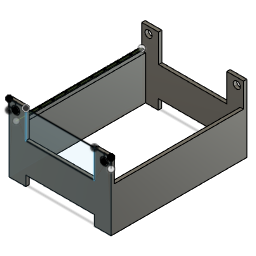
MainBody v5 (Autodesk Fusion 360 design; units mm, degrees)
description: Rack; Circular Pitch: 2.00 mm; Num Teeth: 95; Pressure Angle: 20 deg; Backlash: 0.00 mm;
Autodesk Fusion 360 part; units mm, degrees
note: some values were not read from the file. Set by a fixed rule: which sketch regions a step uses.
sketch "Sketch1" plane through (0, 0, 0) normal (0, 0, 1) x (1, 0, 0)
  line L0 (0, 0) -> (152.4, 0)
  line L1 (152.4, 0) -> (152.4, 101.6)
  line L2 (152.4, 101.6) -> (0, 101.6)
  line L3 (0, 101.6) -> (0, 0)
  line L4 (0, 0) -> (25, 0)
  line L5 (25, 15) -> (25, 0)
  line L6 (152.4, 0) -> (127.4, 0)
  line L7 (127.4, 0) -> (127.4, 15)
  line L8 (127.4, 15) -> (25, 15)
  dimension "d1" = 152.4
  dimension "d2" = 101.6
  dimension "d3" = 25
  constraint horizontal L0
  constraint vertical L1
  constraint horizontal L2
  constraint vertical L3
  constraint coincident L0.start L3.end
  constraint coincident L0 L4.end
  constraint parallel L0 L4
  constraint perpendicular L4 L5
  constraint perpendicular L1 L6
  constraint perpendicular L0 L7
  constraint perpendicular L7 L8
  measures "d1" distance of L0.start L0.end
  measures "d2" distance of L0.start L2.end
  measures "d3" distance of L0.end L6.end
extrude "Extrude1" add sketch "Sketch1" along normal blind 5 contours L0 L1 L2 L3 L4 L5 L6 L7 L8 makes body 1
sketch "Sketch2" plane through (0, 0, 0) normal (0, 0, -1) x (-1, 0, 0)
  line L0 (-152.4, 101.6) -> (-152.4, 0)
  line L1 (-152.4, 0) -> (-127.4, 0)
  line L2 (-127.4, 0) -> (-127.4, 15)
  line L3 (-127.4, 15) -> (-25, 15)
  line L4 (-25, 15) -> (-25, 0)
  line L5 (-25, 0) -> (0, 0)
  line L6 (0, 0) -> (0, 101.6)
  line L7 (0, 101.6) -> (-152.4, 101.6)
  line L8 (-152.4, 0) -> (-147.4, 0)
  line L9 (-147.4, 0) -> (-147.4, 65)
  line L10 (-147.4, 65) -> (-152.4, 65)
  line L11 (-152.4, 65) -> (-152.4, 0)
  line L12 (0, 0) -> (-6, 0)
  line L13 (-6, 0) -> (-6, 65)
  line L14 (-6, 65) -> (0, 65)
  line L15 (0, 65) -> (0, 0)
  dimension "d6" = 5
  dimension "d7" = 65
  dimension "d8" = 6
  dimension "d9" = 65
  constraint horizontal L8
  constraint vertical L9
  constraint horizontal L10
  constraint vertical L11
  constraint coincident L0.end L1.start
  constraint horizontal L12
  constraint vertical L13
  constraint horizontal L14
  constraint vertical L15
  constraint coincident L5.end L6.start
  measures "d6" distance of L0.end L8.end
  measures "d7" distance of L0.end L10.end
  measures "d8" distance of L5.end L12.end
  measures "d9" distance of L5.end L14.end
extrude "Extrude2" add sketch "Sketch2" along normal blind 193.04 contours L0 L1 L8 L9 L10 L11 | L5 L6 L12 L13 L14 L15 bodies 1
sketch "Sketch3" plane through (0, 0, -193.04) normal (0, 0, -1) x (-1, 0, 0)
  line L0 (-152.4, 65) -> (-152.4, 0)
  line L1 (-152.4, 0) -> (-147.4, 0)
  line L2 (-147.4, 0) -> (-147.4, 65)
  line L3 (-147.4, 65) -> (-152.4, 65)
  line L4 (-152.4, 0) -> (-0.3217, 0)
  line L5 (-0.3217, 0) -> (-0.3217, 101.3242)
  line L6 (-0.3217, 101.3242) -> (-152.4, 101.3242)
  line L7 (-152.4, 101.3242) -> (-152.4, 0)
  line L8 (-152.4, 0) -> (-127.4, 0)
  line L9 (-127.4, 0) -> (-127.4, 15)
  line L10 (-127.4, 15) -> (-25, 15)
  line L11 (-25, 15) -> (-25, 0)
  dimension "d12" = 25
  constraint horizontal L4
  constraint vertical L5
  constraint horizontal L6
  constraint vertical L7
  constraint coincident L0.end L1.start
  constraint perpendicular L7 L8
  constraint perpendicular L8 L9
  constraint perpendicular L9 L10
  constraint coincident L4 L11.end
  constraint perpendicular L4 L11
  measures "d12" distance of L0.end L8.end
extrude "Extrude3" add sketch "Sketch3" along normal blind 5 contours L0 L1 L2 L3 L4 L7 L8 | L2 L3 L4 L5 L6 L7 L8 L9 L10 L11 bodies 1
sketch "Sketch4" plane through (152.4, 0, 0) normal (1, 0, 0) x (0, 0, -1)
  line L0 (0, 65) -> (0, 101.6)
  line L1 (0, 101.6) -> (-5, 101.6)
  line L2 (-5, 101.6) -> (-5, 0)
  line L3 (-5, 0) -> (198.04, 0)
  line L4 (198.04, 0) -> (198.04, 101.3242)
  line L5 (198.04, 101.3242) -> (193.04, 101.3242)
  line L6 (193.04, 101.3242) -> (193.04, 65)
  line L7 (193.04, 65) -> (0, 65)
sketch "Sketch1 (2)" plane through (0, 0, 0) normal (0, 0, 1) x (1, 0, 0) in component "Rack; Circular Pitch: 2.00 mm; Num Teeth: 95; Pressure Angle: 20 deg; Backlash: 0.00 mm;"
  line L0 (-0.7839, -0.7853) -> (0, -0.5)
  line L1 (0, -0.5) -> (0.6366, -0.2683)
  line L2 (-0.7839, 0.7853) -> (0, 0.5)
  line L3 (0, 0.5) -> (0.6366, 0.2683)
  line L4 (0.6366, 0.2683) -> (0.6366, -0.2683)
  line L5 (-0.7839, 0.7853) -> (-0.7839, 1)
  line L6 (-0.7839, -0.7853) -> (-0.7839, -1)
  line L7 (-0.7839, 1.2147) -> (0, 1.5)
  line L8 (0, 1.5) -> (0.6366, 1.7317)
  line L9 (-0.7839, 2.7853) -> (0, 2.5)
  line L10 (0, 2.5) -> (0.6366, 2.2683)
  line L11 (0.6366, 2.2683) -> (0.6366, 1.7317)
  line L12 (-0.7839, 2.7853) -> (-0.7839, 3)
  line L13 (-0.7839, 1.2147) -> (-0.7839, 1)
  line L14 (-0.7839, 3.2147) -> (0, 3.5)
  line L15 (0, 3.5) -> (0.6366, 3.7317)
  line L16 (-0.7839, 4.7853) -> (0, 4.5)
  line L17 (0, 4.5) -> (0.6366, 4.2683)
  line L18 (0.6366, 4.2683) -> (0.6366, 3.7317)
  line L19 (-0.7839, 4.7853) -> (-0.7839, 5)
  line L20 (-0.7839, 3.2147) -> (-0.7839, 3)
  line L21 (-0.7839, 5.2147) -> (0, 5.5)
  line L22 (0, 5.5) -> (0.6366, 5.7317)
  line L23 (-0.7839, 6.7853) -> (0, 6.5)
  line L24 (0, 6.5) -> (0.6366, 6.2683)
  line L25 (0.6366, 6.2683) -> (0.6366, 5.7317)
  line L26 (-0.7839, 6.7853) -> (-0.7839, 7)
  line L27 (-0.7839, 5.2147) -> (-0.7839, 5)
  line L28 (-0.7839, 7.2147) -> (0, 7.5)
  line L29 (0, 7.5) -> (0.6366, 7.7317)
  line L30 (-0.7839, 8.7853) -> (0, 8.5)
  line L31 (0, 8.5) -> (0.6366, 8.2683)
  line L32 (0.6366, 8.2683) -> (0.6366, 7.7317)
  line L33 (-0.7839, 8.7853) -> (-0.7839, 9)
  line L34 (-0.7839, 7.2147) -> (-0.7839, 7)
  line L35 (-0.7839, 9.2147) -> (0, 9.5)
  line L36 (0, 9.5) -> (0.6366, 9.7317)
  line L37 (-0.7839, 10.7853) -> (0, 10.5)
  line L38 (0, 10.5) -> (0.6366, 10.2683)
  line L39 (0.6366, 10.2683) -> (0.6366, 9.7317)
  line L40 (-0.7839, 10.7853) -> (-0.7839, 11)
  line L41 (-0.7839, 9.2147) -> (-0.7839, 9)
  line L42 (-0.7839, 11.2147) -> (0, 11.5)
  line L43 (0, 11.5) -> (0.6366, 11.7317)
  line L44 (-0.7839, 12.7853) -> (0, 12.5)
  line L45 (0, 12.5) -> (0.6366, 12.2683)
  line L46 (0.6366, 12.2683) -> (0.6366, 11.7317)
  line L47 (-0.7839, 12.7853) -> (-0.7839, 13)
  line L48 (-0.7839, 11.2147) -> (-0.7839, 11)
  line L49 (-0.7839, 13.2147) -> (0, 13.5)
  line L50 (0, 13.5) -> (0.6366, 13.7317)
  line L51 (-0.7839, 14.7853) -> (0, 14.5)
  line L52 (0, 14.5) -> (0.6366, 14.2683)
  line L53 (0.6366, 14.2683) -> (0.6366, 13.7317)
  line L54 (-0.7839, 14.7853) -> (-0.7839, 15)
  line L55 (-0.7839, 13.2147) -> (-0.7839, 13)
  line L56 (-0.7839, 15.2147) -> (0, 15.5)
  line L57 (0, 15.5) -> (0.6366, 15.7317)
  line L58 (-0.7839, 16.7853) -> (0, 16.5)
  line L59 (0, 16.5) -> (0.6366, 16.2683)
  line L60 (0.6366, 16.2683) -> (0.6366, 15.7317)
  line L61 (-0.7839, 16.7853) -> (-0.7839, 17)
  line L62 (-0.7839, 15.2147) -> (-0.7839, 15)
  line L63 (-0.7839, 17.2147) -> (0, 17.5)
  line L64 (0, 17.5) -> (0.6366, 17.7317)
  line L65 (-0.7839, 18.7853) -> (0, 18.5)
  line L66 (0, 18.5) -> (0.6366, 18.2683)
  line L67 (0.6366, 18.2683) -> (0.6366, 17.7317)
  line L68 (-0.7839, 18.7853) -> (-0.7839, 19)
  line L69 (-0.7839, 17.2147) -> (-0.7839, 17)
  line L70 (-0.7839, 19.2147) -> (0, 19.5)
  line L71 (0, 19.5) -> (0.6366, 19.7317)
  line L72 (-0.7839, 20.7853) -> (0, 20.5)
  line L73 (0, 20.5) -> (0.6366, 20.2683)
  line L74 (0.6366, 20.2683) -> (0.6366, 19.7317)
  line L75 (-0.7839, 20.7853) -> (-0.7839, 21)
  line L76 (-0.7839, 19.2147) -> (-0.7839, 19)
  line L77 (-0.7839, 21.2147) -> (0, 21.5)
  line L78 (0, 21.5) -> (0.6366, 21.7317)
  line L79 (-0.7839, 22.7853) -> (0, 22.5)
  line L80 (0, 22.5) -> (0.6366, 22.2683)
  line L81 (0.6366, 22.2683) -> (0.6366, 21.7317)
  line L82 (-0.7839, 22.7853) -> (-0.7839, 23)
  line L83 (-0.7839, 21.2147) -> (-0.7839, 21)
  line L84 (-0.7839, 23.2147) -> (0, 23.5)
  line L85 (0, 23.5) -> (0.6366, 23.7317)
  line L86 (-0.7839, 24.7853) -> (0, 24.5)
  line L87 (0, 24.5) -> (0.6366, 24.2683)
  line L88 (0.6366, 24.2683) -> (0.6366, 23.7317)
  line L89 (-0.7839, 24.7853) -> (-0.7839, 25)
  line L90 (-0.7839, 23.2147) -> (-0.7839, 23)
  line L91 (-0.7839, 25.2147) -> (0, 25.5)
  line L92 (0, 25.5) -> (0.6366, 25.7317)
  line L93 (-0.7839, 26.7853) -> (0, 26.5)
  line L94 (0, 26.5) -> (0.6366, 26.2683)
  line L95 (0.6366, 26.2683) -> (0.6366, 25.7317)
  line L96 (-0.7839, 26.7853) -> (-0.7839, 27)
  line L97 (-0.7839, 25.2147) -> (-0.7839, 25)
  line L98 (-0.7839, 27.2147) -> (0, 27.5)
  line L99 (0, 27.5) -> (0.6366, 27.7317)
  line L100 (-0.7839, 28.7853) -> (0, 28.5)
  line L101 (0, 28.5) -> (0.6366, 28.2683)
  line L102 (0.6366, 28.2683) -> (0.6366, 27.7317)
  line L103 (-0.7839, 28.7853) -> (-0.7839, 29)
  line L104 (-0.7839, 27.2147) -> (-0.7839, 27)
  line L105 (-0.7839, 29.2147) -> (0, 29.5)
  line L106 (0, 29.5) -> (0.6366, 29.7317)
  line L107 (-0.7839, 30.7853) -> (0, 30.5)
  line L108 (0, 30.5) -> (0.6366, 30.2683)
  line L109 (0.6366, 30.2683) -> (0.6366, 29.7317)
  line L110 (-0.7839, 30.7853) -> (-0.7839, 31)
  line L111 (-0.7839, 29.2147) -> (-0.7839, 29)
  line L112 (-0.7839, 31.2147) -> (0, 31.5)
  line L113 (0, 31.5) -> (0.6366, 31.7317)
  line L114 (-0.7839, 32.7853) -> (0, 32.5)
  line L115 (0, 32.5) -> (0.6366, 32.2683)
  line L116 (0.6366, 32.2683) -> (0.6366, 31.7317)
  line L117 (-0.7839, 32.7853) -> (-0.7839, 33)
  line L118 (-0.7839, 31.2147) -> (-0.7839, 31)
  line L119 (-0.7839, 33.2147) -> (0, 33.5)
  line L120 (0, 33.5) -> (0.6366, 33.7317)
  line L121 (-0.7839, 34.7853) -> (0, 34.5)
  line L122 (0, 34.5) -> (0.6366, 34.2683)
  line L123 (0.6366, 34.2683) -> (0.6366, 33.7317)
  line L124 (-0.7839, 34.7853) -> (-0.7839, 35)
  line L125 (-0.7839, 33.2147) -> (-0.7839, 33)
  line L126 (-0.7839, 35.2147) -> (0, 35.5)
  line L127 (0, 35.5) -> (0.6366, 35.7317)
  line L128 (-0.7839, 36.7853) -> (0, 36.5)
  line L129 (0, 36.5) -> (0.6366, 36.2683)
  line L130 (0.6366, 36.2683) -> (0.6366, 35.7317)
  line L131 (-0.7839, 36.7853) -> (-0.7839, 37)
  line L132 (-0.7839, 35.2147) -> (-0.7839, 35)
  line L133 (-0.7839, 37.2147) -> (0, 37.5)
  line L134 (0, 37.5) -> (0.6366, 37.7317)
  line L135 (-0.7839, 38.7853) -> (0, 38.5)
  line L136 (0, 38.5) -> (0.6366, 38.2683)
  line L137 (0.6366, 38.2683) -> (0.6366, 37.7317)
  line L138 (-0.7839, 38.7853) -> (-0.7839, 39)
  line L139 (-0.7839, 37.2147) -> (-0.7839, 37)
  line L140 (-0.7839, 39.2147) -> (0, 39.5)
  line L141 (0, 39.5) -> (0.6366, 39.7317)
  line L142 (-0.7839, 40.7853) -> (0, 40.5)
  line L143 (0, 40.5) -> (0.6366, 40.2683)
  line L144 (0.6366, 40.2683) -> (0.6366, 39.7317)
  line L145 (-0.7839, 40.7853) -> (-0.7839, 41)
  line L146 (-0.7839, 39.2147) -> (-0.7839, 39)
  line L147 (-0.7839, 41.2147) -> (0, 41.5)
  line L148 (0, 41.5) -> (0.6366, 41.7317)
  line L149 (-0.7839, 42.7853) -> (0, 42.5)
  line L150 (0, 42.5) -> (0.6366, 42.2683)
  line L151 (0.6366, 42.2683) -> (0.6366, 41.7317)
  line L152 (-0.7839, 42.7853) -> (-0.7839, 43)
  line L153 (-0.7839, 41.2147) -> (-0.7839, 41)
  line L154 (-0.7839, 43.2147) -> (0, 43.5)
  line L155 (0, 43.5) -> (0.6366, 43.7317)
  line L156 (-0.7839, 44.7853) -> (0, 44.5)
  line L157 (0, 44.5) -> (0.6366, 44.2683)
  line L158 (0.6366, 44.2683) -> (0.6366, 43.7317)
  line L159 (-0.7839, 44.7853) -> (-0.7839, 45)
  line L160 (-0.7839, 43.2147) -> (-0.7839, 43)
  line L161 (-0.7839, 45.2147) -> (0, 45.5)
  line L162 (0, 45.5) -> (0.6366, 45.7317)
  line L163 (-0.7839, 46.7853) -> (0, 46.5)
  line L164 (0, 46.5) -> (0.6366, 46.2683)
  line L165 (0.6366, 46.2683) -> (0.6366, 45.7317)
  line L166 (-0.7839, 46.7853) -> (-0.7839, 47)
  line L167 (-0.7839, 45.2147) -> (-0.7839, 45)
  line L168 (-0.7839, 47.2147) -> (0, 47.5)
  line L169 (0, 47.5) -> (0.6366, 47.7317)
  line L170 (-0.7839, 48.7853) -> (0, 48.5)
  line L171 (0, 48.5) -> (0.6366, 48.2683)
  line L172 (0.6366, 48.2683) -> (0.6366, 47.7317)
  line L173 (-0.7839, 48.7853) -> (-0.7839, 49)
  line L174 (-0.7839, 47.2147) -> (-0.7839, 47)
  line L175 (-0.7839, 49.2147) -> (0, 49.5)
  line L176 (0, 49.5) -> (0.6366, 49.7317)
  line L177 (-0.7839, 50.7853) -> (0, 50.5)
  line L178 (0, 50.5) -> (0.6366, 50.2683)
  line L179 (0.6366, 50.2683) -> (0.6366, 49.7317)
  line L180 (-0.7839, 50.7853) -> (-0.7839, 51)
  line L181 (-0.7839, 49.2147) -> (-0.7839, 49)
  line L182 (-0.7839, 51.2147) -> (0, 51.5)
  line L183 (0, 51.5) -> (0.6366, 51.7317)
  line L184 (-0.7839, 52.7853) -> (0, 52.5)
  line L185 (0, 52.5) -> (0.6366, 52.2683)
  line L186 (0.6366, 52.2683) -> (0.6366, 51.7317)
  line L187 (-0.7839, 52.7853) -> (-0.7839, 53)
  line L188 (-0.7839, 51.2147) -> (-0.7839, 51)
  line L189 (-0.7839, 53.2147) -> (0, 53.5)
  line L190 (0, 53.5) -> (0.6366, 53.7317)
  line L191 (-0.7839, 54.7853) -> (0, 54.5)
  line L192 (0, 54.5) -> (0.6366, 54.2683)
  line L193 (0.6366, 54.2683) -> (0.6366, 53.7317)
  line L194 (-0.7839, 54.7853) -> (-0.7839, 55)
  line L195 (-0.7839, 53.2147) -> (-0.7839, 53)
  line L196 (-0.7839, 55.2147) -> (0, 55.5)
  line L197 (0, 55.5) -> (0.6366, 55.7317)
  line L198 (-0.7839, 56.7853) -> (0, 56.5)
  line L199 (0, 56.5) -> (0.6366, 56.2683)
  line L200 (0.6366, 56.2683) -> (0.6366, 55.7317)
  line L201 (-0.7839, 56.7853) -> (-0.7839, 57)
  line L202 (-0.7839, 55.2147) -> (-0.7839, 55)
  line L203 (-0.7839, 57.2147) -> (0, 57.5)
  line L204 (0, 57.5) -> (0.6366, 57.7317)
  line L205 (-0.7839, 58.7853) -> (0, 58.5)
  line L206 (0, 58.5) -> (0.6366, 58.2683)
  line L207 (0.6366, 58.2683) -> (0.6366, 57.7317)
  line L208 (-0.7839, 58.7853) -> (-0.7839, 59)
  line L209 (-0.7839, 57.2147) -> (-0.7839, 57)
  line L210 (-0.7839, 59.2147) -> (0, 59.5)
  line L211 (0, 59.5) -> (0.6366, 59.7317)
  line L212 (-0.7839, 60.7853) -> (0, 60.5)
  line L213 (0, 60.5) -> (0.6366, 60.2683)
  line L214 (0.6366, 60.2683) -> (0.6366, 59.7317)
  line L215 (-0.7839, 60.7853) -> (-0.7839, 61)
  line L216 (-0.7839, 59.2147) -> (-0.7839, 59)
  line L217 (-0.7839, 61.2147) -> (0, 61.5)
  line L218 (0, 61.5) -> (0.6366, 61.7317)
  line L219 (-0.7839, 62.7853) -> (0, 62.5)
  line L220 (0, 62.5) -> (0.6366, 62.2683)
  line L221 (0.6366, 62.2683) -> (0.6366, 61.7317)
  line L222 (-0.7839, 62.7853) -> (-0.7839, 63)
  line L223 (-0.7839, 61.2147) -> (-0.7839, 61)
  line L224 (-0.7839, 63.2147) -> (0, 63.5)
  line L225 (0, 63.5) -> (0.6366, 63.7317)
  line L226 (-0.7839, 64.7853) -> (0, 64.5)
  line L227 (0, 64.5) -> (0.6366, 64.2683)
  line L228 (0.6366, 64.2683) -> (0.6366, 63.7317)
  line L229 (-0.7839, 64.7853) -> (-0.7839, 65)
  line L230 (-0.7839, 63.2147) -> (-0.7839, 63)
  line L231 (-0.7839, 65.2147) -> (0, 65.5)
  line L232 (0, 65.5) -> (0.6366, 65.7317)
  line L233 (-0.7839, 66.7853) -> (0, 66.5)
  line L234 (0, 66.5) -> (0.6366, 66.2683)
  line L235 (0.6366, 66.2683) -> (0.6366, 65.7317)
  line L236 (-0.7839, 66.7853) -> (-0.7839, 67)
  line L237 (-0.7839, 65.2147) -> (-0.7839, 65)
  line L238 (-0.7839, 67.2147) -> (0, 67.5)
  line L239 (0, 67.5) -> (0.6366, 67.7317)
  line L240 (-0.7839, 68.7853) -> (0, 68.5)
  line L241 (0, 68.5) -> (0.6366, 68.2683)
  line L242 (0.6366, 68.2683) -> (0.6366, 67.7317)
  line L243 (-0.7839, 68.7853) -> (-0.7839, 69)
  line L244 (-0.7839, 67.2147) -> (-0.7839, 67)
  line L245 (-0.7839, 69.2147) -> (0, 69.5)
  line L246 (0, 69.5) -> (0.6366, 69.7317)
  line L247 (-0.7839, 70.7853) -> (0, 70.5)
  line L248 (0, 70.5) -> (0.6366, 70.2683)
  line L249 (0.6366, 70.2683) -> (0.6366, 69.7317)
  line L250 (-0.7839, 70.7853) -> (-0.7839, 71)
  line L251 (-0.7839, 69.2147) -> (-0.7839, 69)
  line L252 (-0.7839, 71.2147) -> (0, 71.5)
  line L253 (0, 71.5) -> (0.6366, 71.7317)
  line L254 (-0.7839, 72.7853) -> (0, 72.5)
  line L255 (0, 72.5) -> (0.6366, 72.2683)
  line L256 (0.6366, 72.2683) -> (0.6366, 71.7317)
  line L257 (-0.7839, 72.7853) -> (-0.7839, 73)
  line L258 (-0.7839, 71.2147) -> (-0.7839, 71)
  line L259 (-0.7839, 73.2147) -> (0, 73.5)
  line L260 (0, 73.5) -> (0.6366, 73.7317)
  line L261 (-0.7839, 74.7853) -> (0, 74.5)
  line L262 (0, 74.5) -> (0.6366, 74.2683)
  line L263 (0.6366, 74.2683) -> (0.6366, 73.7317)
  line L264 (-0.7839, 74.7853) -> (-0.7839, 75)
  line L265 (-0.7839, 73.2147) -> (-0.7839, 73)
  line L266 (-0.7839, 75.2147) -> (0, 75.5)
  line L267 (0, 75.5) -> (0.6366, 75.7317)
  line L268 (-0.7839, 76.7853) -> (0, 76.5)
  line L269 (0, 76.5) -> (0.6366, 76.2683)
  line L270 (0.6366, 76.2683) -> (0.6366, 75.7317)
  line L271 (-0.7839, 76.7853) -> (-0.7839, 77)
  line L272 (-0.7839, 75.2147) -> (-0.7839, 75)
  line L273 (-0.7839, 77.2147) -> (0, 77.5)
  line L274 (0, 77.5) -> (0.6366, 77.7317)
  line L275 (-0.7839, 78.7853) -> (0, 78.5)
  line L276 (0, 78.5) -> (0.6366, 78.2683)
  line L277 (0.6366, 78.2683) -> (0.6366, 77.7317)
  line L278 (-0.7839, 78.7853) -> (-0.7839, 79)
  line L279 (-0.7839, 77.2147) -> (-0.7839, 77)
  line L280 (-0.7839, 79.2147) -> (0, 79.5)
  line L281 (0, 79.5) -> (0.6366, 79.7317)
  line L282 (-0.7839, 80.7853) -> (0, 80.5)
  line L283 (0, 80.5) -> (0.6366, 80.2683)
  line L284 (0.6366, 80.2683) -> (0.6366, 79.7317)
  line L285 (-0.7839, 80.7853) -> (-0.7839, 81)
  line L286 (-0.7839, 79.2147) -> (-0.7839, 79)
  line L287 (-0.7839, 81.2147) -> (0, 81.5)
  line L288 (0, 81.5) -> (0.6366, 81.7317)
  line L289 (-0.7839, 82.7853) -> (0, 82.5)
  line L290 (0, 82.5) -> (0.6366, 82.2683)
  line L291 (0.6366, 82.2683) -> (0.6366, 81.7317)
  line L292 (-0.7839, 82.7853) -> (-0.7839, 83)
  line L293 (-0.7839, 81.2147) -> (-0.7839, 81)
  line L294 (-0.7839, 83.2147) -> (0, 83.5)
  line L295 (0, 83.5) -> (0.6366, 83.7317)
  line L296 (-0.7839, 84.7853) -> (0, 84.5)
  line L297 (0, 84.5) -> (0.6366, 84.2683)
  line L298 (0.6366, 84.2683) -> (0.6366, 83.7317)
  line L299 (-0.7839, 84.7853) -> (-0.7839, 85)
  line L300 (-0.7839, 83.2147) -> (-0.7839, 83)
  line L301 (-0.7839, 85.2147) -> (0, 85.5)
  line L302 (0, 85.5) -> (0.6366, 85.7317)
  line L303 (-0.7839, 86.7853) -> (0, 86.5)
  line L304 (0, 86.5) -> (0.6366, 86.2683)
  line L305 (0.6366, 86.2683) -> (0.6366, 85.7317)
  line L306 (-0.7839, 86.7853) -> (-0.7839, 87)
  line L307 (-0.7839, 85.2147) -> (-0.7839, 85)
  line L308 (-0.7839, 87.2147) -> (0, 87.5)
  line L309 (0, 87.5) -> (0.6366, 87.7317)
  line L310 (-0.7839, 88.7853) -> (0, 88.5)
  line L311 (0, 88.5) -> (0.6366, 88.2683)
  line L312 (0.6366, 88.2683) -> (0.6366, 87.7317)
  line L313 (-0.7839, 88.7853) -> (-0.7839, 89)
  line L314 (-0.7839, 87.2147) -> (-0.7839, 87)
  line L315 (-0.7839, 89.2147) -> (0, 89.5)
  line L316 (0, 89.5) -> (0.6366, 89.7317)
  line L317 (-0.7839, 90.7853) -> (0, 90.5)
  line L318 (0, 90.5) -> (0.6366, 90.2683)
  line L319 (0.6366, 90.2683) -> (0.6366, 89.7317)
  line L320 (-0.7839, 90.7853) -> (-0.7839, 91)
  line L321 (-0.7839, 89.2147) -> (-0.7839, 89)
  line L322 (-0.7839, 91.2147) -> (0, 91.5)
  line L323 (0, 91.5) -> (0.6366, 91.7317)
  line L324 (-0.7839, 92.7853) -> (0, 92.5)
  line L325 (0, 92.5) -> (0.6366, 92.2683)
  line L326 (0.6366, 92.2683) -> (0.6366, 91.7317)
  line L327 (-0.7839, 92.7853) -> (-0.7839, 93)
  line L328 (-0.7839, 91.2147) -> (-0.7839, 91)
  line L329 (-0.7839, 93.2147) -> (0, 93.5)
  line L330 (0, 93.5) -> (0.6366, 93.7317)
  line L331 (-0.7839, 94.7853) -> (0, 94.5)
  line L332 (0, 94.5) -> (0.6366, 94.2683)
  line L333 (0.6366, 94.2683) -> (0.6366, 93.7317)
  line L334 (-0.7839, 94.7853) -> (-0.7839, 95)
  line L335 (-0.7839, 93.2147) -> (-0.7839, 93)
  line L336 (-0.7839, 95.2147) -> (0, 95.5)
  line L337 (0, 95.5) -> (0.6366, 95.7317)
  line L338 (-0.7839, 96.7853) -> (0, 96.5)
  line L339 (0, 96.5) -> (0.6366, 96.2683)
  line L340 (0.6366, 96.2683) -> (0.6366, 95.7317)
  line L341 (-0.7839, 96.7853) -> (-0.7839, 97)
  line L342 (-0.7839, 95.2147) -> (-0.7839, 95)
  line L343 (-0.7839, 97.2147) -> (0, 97.5)
  line L344 (0, 97.5) -> (0.6366, 97.7317)
  line L345 (-0.7839, 98.7853) -> (0, 98.5)
  line L346 (0, 98.5) -> (0.6366, 98.2683)
  line L347 (0.6366, 98.2683) -> (0.6366, 97.7317)
  line L348 (-0.7839, 98.7853) -> (-0.7839, 99)
  line L349 (-0.7839, 97.2147) -> (-0.7839, 97)
  line L350 (-0.7839, 99.2147) -> (0, 99.5)
  line L351 (0, 99.5) -> (0.6366, 99.7317)
  line L352 (-0.7839, 100.7853) -> (0, 100.5)
  line L353 (0, 100.5) -> (0.6366, 100.2683)
  line L354 (0.6366, 100.2683) -> (0.6366, 99.7317)
  line L355 (-0.7839, 100.7853) -> (-0.7839, 101)
  line L356 (-0.7839, 99.2147) -> (-0.7839, 99)
  line L357 (-0.7839, 101.2147) -> (0, 101.5)
  line L358 (0, 101.5) -> (0.6366, 101.7317)
  line L359 (-0.7839, 102.7853) -> (0, 102.5)
  line L360 (0, 102.5) -> (0.6366, 102.2683)
  line L361 (0.6366, 102.2683) -> (0.6366, 101.7317)
  line L362 (-0.7839, 102.7853) -> (-0.7839, 103)
  line L363 (-0.7839, 101.2147) -> (-0.7839, 101)
  line L364 (-0.7839, 103.2147) -> (0, 103.5)
  line L365 (0, 103.5) -> (0.6366, 103.7317)
  line L366 (-0.7839, 104.7853) -> (0, 104.5)
  line L367 (0, 104.5) -> (0.6366, 104.2683)
  line L368 (0.6366, 104.2683) -> (0.6366, 103.7317)
  line L369 (-0.7839, 104.7853) -> (-0.7839, 105)
  line L370 (-0.7839, 103.2147) -> (-0.7839, 103)
  line L371 (-0.7839, 105.2147) -> (0, 105.5)
  line L372 (0, 105.5) -> (0.6366, 105.7317)
  line L373 (-0.7839, 106.7853) -> (0, 106.5)
  line L374 (0, 106.5) -> (0.6366, 106.2683)
  line L375 (0.6366, 106.2683) -> (0.6366, 105.7317)
  line L376 (-0.7839, 106.7853) -> (-0.7839, 107)
  line L377 (-0.7839, 105.2147) -> (-0.7839, 105)
  line L378 (-0.7839, 107.2147) -> (0, 107.5)
  line L379 (0, 107.5) -> (0.6366, 107.7317)
  line L380 (-0.7839, 108.7853) -> (0, 108.5)
  line L381 (0, 108.5) -> (0.6366, 108.2683)
  line L382 (0.6366, 108.2683) -> (0.6366, 107.7317)
  line L383 (-0.7839, 108.7853) -> (-0.7839, 109)
  line L384 (-0.7839, 107.2147) -> (-0.7839, 107)
  line L385 (-0.7839, 109.2147) -> (0, 109.5)
  line L386 (0, 109.5) -> (0.6366, 109.7317)
  line L387 (-0.7839, 110.7853) -> (0, 110.5)
  line L388 (0, 110.5) -> (0.6366, 110.2683)
  line L389 (0.6366, 110.2683) -> (0.6366, 109.7317)
  line L390 (-0.7839, 110.7853) -> (-0.7839, 111)
  line L391 (-0.7839, 109.2147) -> (-0.7839, 109)
  line L392 (-0.7839, 111.2147) -> (0, 111.5)
  line L393 (0, 111.5) -> (0.6366, 111.7317)
  line L394 (-0.7839, 112.7853) -> (0, 112.5)
  line L395 (0, 112.5) -> (0.6366, 112.2683)
  line L396 (0.6366, 112.2683) -> (0.6366, 111.7317)
  line L397 (-0.7839, 112.7853) -> (-0.7839, 113)
  line L398 (-0.7839, 111.2147) -> (-0.7839, 111)
  line L399 (-0.7839, 113.2147) -> (0, 113.5)
  line L400 (0, 113.5) -> (0.6366, 113.7317)
  line L401 (-0.7839, 114.7853) -> (0, 114.5)
  line L402 (0, 114.5) -> (0.6366, 114.2683)
  line L403 (0.6366, 114.2683) -> (0.6366, 113.7317)
  line L404 (-0.7839, 114.7853) -> (-0.7839, 115)
  line L405 (-0.7839, 113.2147) -> (-0.7839, 113)
  line L406 (-0.7839, 115.2147) -> (0, 115.5)
  line L407 (0, 115.5) -> (0.6366, 115.7317)
  line L408 (-0.7839, 116.7853) -> (0, 116.5)
  line L409 (0, 116.5) -> (0.6366, 116.2683)
  line L410 (0.6366, 116.2683) -> (0.6366, 115.7317)
  line L411 (-0.7839, 116.7853) -> (-0.7839, 117)
  line L412 (-0.7839, 115.2147) -> (-0.7839, 115)
  line L413 (-0.7839, 117.2147) -> (0, 117.5)
  line L414 (0, 117.5) -> (0.6366, 117.7317)
  line L415 (-0.7839, 118.7853) -> (0, 118.5)
  line L416 (0, 118.5) -> (0.6366, 118.2683)
  line L417 (0.6366, 118.2683) -> (0.6366, 117.7317)
  line L418 (-0.7839, 118.7853) -> (-0.7839, 119)
  line L419 (-0.7839, 117.2147) -> (-0.7839, 117)
  line L420 (-0.7839, 119.2147) -> (0, 119.5)
  line L421 (0, 119.5) -> (0.6366, 119.7317)
  line L422 (-0.7839, 120.7853) -> (0, 120.5)
  line L423 (0, 120.5) -> (0.6366, 120.2683)
  line L424 (0.6366, 120.2683) -> (0.6366, 119.7317)
  line L425 (-0.7839, 120.7853) -> (-0.7839, 121)
  line L426 (-0.7839, 119.2147) -> (-0.7839, 119)
  line L427 (-0.7839, 121.2147) -> (0, 121.5)
  line L428 (0, 121.5) -> (0.6366, 121.7317)
  line L429 (-0.7839, 122.7853) -> (0, 122.5)
  line L430 (0, 122.5) -> (0.6366, 122.2683)
  line L431 (0.6366, 122.2683) -> (0.6366, 121.7317)
  line L432 (-0.7839, 122.7853) -> (-0.7839, 123)
  line L433 (-0.7839, 121.2147) -> (-0.7839, 121)
  line L434 (-0.7839, 123.2147) -> (0, 123.5)
  line L435 (0, 123.5) -> (0.6366, 123.7317)
  line L436 (-0.7839, 124.7853) -> (0, 124.5)
  line L437 (0, 124.5) -> (0.6366, 124.2683)
  line L438 (0.6366, 124.2683) -> (0.6366, 123.7317)
  line L439 (-0.7839, 124.7853) -> (-0.7839, 125)
  line L440 (-0.7839, 123.2147) -> (-0.7839, 123)
  line L441 (-0.7839, 125.2147) -> (0, 125.5)
  line L442 (0, 125.5) -> (0.6366, 125.7317)
  line L443 (-0.7839, 126.7853) -> (0, 126.5)
  line L444 (0, 126.5) -> (0.6366, 126.2683)
  line L445 (0.6366, 126.2683) -> (0.6366, 125.7317)
  line L446 (-0.7839, 126.7853) -> (-0.7839, 127)
  line L447 (-0.7839, 125.2147) -> (-0.7839, 125)
  line L448 (-0.7839, 127.2147) -> (0, 127.5)
  line L449 (0, 127.5) -> (0.6366, 127.7317)
  line L450 (-0.7839, 128.7853) -> (0, 128.5)
  line L451 (0, 128.5) -> (0.6366, 128.2683)
  line L452 (0.6366, 128.2683) -> (0.6366, 127.7317)
  line L453 (-0.7839, 128.7853) -> (-0.7839, 129)
  line L454 (-0.7839, 127.2147) -> (-0.7839, 127)
  line L455 (-0.7839, 129.2147) -> (0, 129.5)
  line L456 (0, 129.5) -> (0.6366, 129.7317)
  line L457 (-0.7839, 130.7853) -> (0, 130.5)
  line L458 (0, 130.5) -> (0.6366, 130.2683)
  line L459 (0.6366, 130.2683) -> (0.6366, 129.7317)
  line L460 (-0.7839, 130.7853) -> (-0.7839, 131)
  line L461 (-0.7839, 129.2147) -> (-0.7839, 129)
  line L462 (-0.7839, 131.2147) -> (0, 131.5)
  line L463 (0, 131.5) -> (0.6366, 131.7317)
  line L464 (-0.7839, 132.7853) -> (0, 132.5)
  line L465 (0, 132.5) -> (0.6366, 132.2683)
  line L466 (0.6366, 132.2683) -> (0.6366, 131.7317)
  line L467 (-0.7839, 132.7853) -> (-0.7839, 133)
  line L468 (-0.7839, 131.2147) -> (-0.7839, 131)
  line L469 (-0.7839, 133.2147) -> (0, 133.5)
  line L470 (0, 133.5) -> (0.6366, 133.7317)
  line L471 (-0.7839, 134.7853) -> (0, 134.5)
  line L472 (0, 134.5) -> (0.6366, 134.2683)
  line L473 (0.6366, 134.2683) -> (0.6366, 133.7317)
  line L474 (-0.7839, 134.7853) -> (-0.7839, 135)
  line L475 (-0.7839, 133.2147) -> (-0.7839, 133)
  line L476 (-0.7839, 135.2147) -> (0, 135.5)
  line L477 (0, 135.5) -> (0.6366, 135.7317)
  line L478 (-0.7839, 136.7853) -> (0, 136.5)
  line L479 (0, 136.5) -> (0.6366, 136.2683)
  line L480 (0.6366, 136.2683) -> (0.6366, 135.7317)
  line L481 (-0.7839, 136.7853) -> (-0.7839, 137)
  line L482 (-0.7839, 135.2147) -> (-0.7839, 135)
  line L483 (-0.7839, 137.2147) -> (0, 137.5)
  line L484 (0, 137.5) -> (0.6366, 137.7317)
  line L485 (-0.7839, 138.7853) -> (0, 138.5)
  line L486 (0, 138.5) -> (0.6366, 138.2683)
  line L487 (0.6366, 138.2683) -> (0.6366, 137.7317)
  line L488 (-0.7839, 138.7853) -> (-0.7839, 139)
  line L489 (-0.7839, 137.2147) -> (-0.7839, 137)
  line L490 (-0.7839, 139.2147) -> (0, 139.5)
  line L491 (0, 139.5) -> (0.6366, 139.7317)
  line L492 (-0.7839, 140.7853) -> (0, 140.5)
  line L493 (0, 140.5) -> (0.6366, 140.2683)
  line L494 (0.6366, 140.2683) -> (0.6366, 139.7317)
  line L495 (-0.7839, 140.7853) -> (-0.7839, 141)
  line L496 (-0.7839, 139.2147) -> (-0.7839, 139)
  line L497 (-0.7839, 141.2147) -> (0, 141.5)
  line L498 (0, 141.5) -> (0.6366, 141.7317)
  line L499 (-0.7839, 142.7853) -> (0, 142.5)
  line L500 (0, 142.5) -> (0.6366, 142.2683)
  line L501 (0.6366, 142.2683) -> (0.6366, 141.7317)
  line L502 (-0.7839, 142.7853) -> (-0.7839, 143)
  line L503 (-0.7839, 141.2147) -> (-0.7839, 141)
  line L504 (-0.7839, 143.2147) -> (0, 143.5)
  line L505 (0, 143.5) -> (0.6366, 143.7317)
  line L506 (-0.7839, 144.7853) -> (0, 144.5)
  line L507 (0, 144.5) -> (0.6366, 144.2683)
  line L508 (0.6366, 144.2683) -> (0.6366, 143.7317)
  line L509 (-0.7839, 144.7853) -> (-0.7839, 145)
  line L510 (-0.7839, 143.2147) -> (-0.7839, 143)
  line L511 (-0.7839, 145.2147) -> (0, 145.5)
  line L512 (0, 145.5) -> (0.6366, 145.7317)
  line L513 (-0.7839, 146.7853) -> (0, 146.5)
  line L514 (0, 146.5) -> (0.6366, 146.2683)
  line L515 (0.6366, 146.2683) -> (0.6366, 145.7317)
  line L516 (-0.7839, 146.7853) -> (-0.7839, 147)
  line L517 (-0.7839, 145.2147) -> (-0.7839, 145)
  line L518 (-0.7839, 147.2147) -> (0, 147.5)
  line L519 (0, 147.5) -> (0.6366, 147.7317)
  line L520 (-0.7839, 148.7853) -> (0, 148.5)
  line L521 (0, 148.5) -> (0.6366, 148.2683)
  line L522 (0.6366, 148.2683) -> (0.6366, 147.7317)
  line L523 (-0.7839, 148.7853) -> (-0.7839, 149)
  line L524 (-0.7839, 147.2147) -> (-0.7839, 147)
  line L525 (-0.7839, 149.2147) -> (0, 149.5)
  line L526 (0, 149.5) -> (0.6366, 149.7317)
  line L527 (-0.7839, 150.7853) -> (0, 150.5)
  line L528 (0, 150.5) -> (0.6366, 150.2683)
  line L529 (0.6366, 150.2683) -> (0.6366, 149.7317)
  line L530 (-0.7839, 150.7853) -> (-0.7839, 151)
  line L531 (-0.7839, 149.2147) -> (-0.7839, 149)
  line L532 (-0.7839, 151.2147) -> (0, 151.5)
  line L533 (0, 151.5) -> (0.6366, 151.7317)
  line L534 (-0.7839, 152.7853) -> (0, 152.5)
  line L535 (0, 152.5) -> (0.6366, 152.2683)
  line L536 (0.6366, 152.2683) -> (0.6366, 151.7317)
  line L537 (-0.7839, 152.7853) -> (-0.7839, 153)
  line L538 (-0.7839, 151.2147) -> (-0.7839, 151)
  line L539 (-0.7839, 153.2147) -> (0, 153.5)
  line L540 (0, 153.5) -> (0.6366, 153.7317)
  line L541 (-0.7839, 154.7853) -> (0, 154.5)
  line L542 (0, 154.5) -> (0.6366, 154.2683)
  line L543 (0.6366, 154.2683) -> (0.6366, 153.7317)
  line L544 (-0.7839, 154.7853) -> (-0.7839, 155)
  line L545 (-0.7839, 153.2147) -> (-0.7839, 153)
  line L546 (-0.7839, 155.2147) -> (0, 155.5)
  line L547 (0, 155.5) -> (0.6366, 155.7317)
  line L548 (-0.7839, 156.7853) -> (0, 156.5)
  line L549 (0, 156.5) -> (0.6366, 156.2683)
  line L550 (0.6366, 156.2683) -> (0.6366, 155.7317)
  line L551 (-0.7839, 156.7853) -> (-0.7839, 157)
  line L552 (-0.7839, 155.2147) -> (-0.7839, 155)
  line L553 (-0.7839, 157.2147) -> (0, 157.5)
  line L554 (0, 157.5) -> (0.6366, 157.7317)
  line L555 (-0.7839, 158.7853) -> (0, 158.5)
  line L556 (0, 158.5) -> (0.6366, 158.2683)
  line L557 (0.6366, 158.2683) -> (0.6366, 157.7317)
  line L558 (-0.7839, 158.7853) -> (-0.7839, 159)
  line L559 (-0.7839, 157.2147) -> (-0.7839, 157)
  line L560 (-0.7839, 159.2147) -> (0, 159.5)
  line L561 (0, 159.5) -> (0.6366, 159.7317)
  line L562 (-0.7839, 160.7853) -> (0, 160.5)
  line L563 (0, 160.5) -> (0.6366, 160.2683)
  line L564 (0.6366, 160.2683) -> (0.6366, 159.7317)
  line L565 (-0.7839, 160.7853) -> (-0.7839, 161)
  line L566 (-0.7839, 159.2147) -> (-0.7839, 159)
  line L567 (-0.7839, 161.2147) -> (0, 161.5)
  line L568 (0, 161.5) -> (0.6366, 161.7317)
  line L569 (-0.7839, 162.7853) -> (0, 162.5)
  line L570 (0, 162.5) -> (0.6366, 162.2683)
  line L571 (0.6366, 162.2683) -> (0.6366, 161.7317)
  line L572 (-0.7839, 162.7853) -> (-0.7839, 163)
  line L573 (-0.7839, 161.2147) -> (-0.7839, 161)
  line L574 (-0.7839, 163.2147) -> (0, 163.5)
  line L575 (0, 163.5) -> (0.6366, 163.7317)
  line L576 (-0.7839, 164.7853) -> (0, 164.5)
  line L577 (0, 164.5) -> (0.6366, 164.2683)
  line L578 (0.6366, 164.2683) -> (0.6366, 163.7317)
  line L579 (-0.7839, 164.7853) -> (-0.7839, 165)
  line L580 (-0.7839, 163.2147) -> (-0.7839, 163)
  line L581 (-0.7839, 165.2147) -> (0, 165.5)
  line L582 (0, 165.5) -> (0.6366, 165.7317)
  line L583 (-0.7839, 166.7853) -> (0, 166.5)
  line L584 (0, 166.5) -> (0.6366, 166.2683)
  line L585 (0.6366, 166.2683) -> (0.6366, 165.7317)
  line L586 (-0.7839, 166.7853) -> (-0.7839, 167)
  line L587 (-0.7839, 165.2147) -> (-0.7839, 165)
  line L588 (-0.7839, 167.2147) -> (0, 167.5)
  line L589 (0, 167.5) -> (0.6366, 167.7317)
  line L590 (-0.7839, 168.7853) -> (0, 168.5)
  line L591 (0, 168.5) -> (0.6366, 168.2683)
  line L592 (0.6366, 168.2683) -> (0.6366, 167.7317)
  line L593 (-0.7839, 168.7853) -> (-0.7839, 169)
  line L594 (-0.7839, 167.2147) -> (-0.7839, 167)
  line L595 (-0.7839, 169.2147) -> (0, 169.5)
  line L596 (0, 169.5) -> (0.6366, 169.7317)
  line L597 (-0.7839, 170.7853) -> (0, 170.5)
  line L598 (0, 170.5) -> (0.6366, 170.2683)
  line L599 (0.6366, 170.2683) -> (0.6366, 169.7317)
  line L600 (-0.7839, 170.7853) -> (-0.7839, 171)
  line L601 (-0.7839, 169.2147) -> (-0.7839, 169)
  line L602 (-0.7839, 171.2147) -> (0, 171.5)
  line L603 (0, 171.5) -> (0.6366, 171.7317)
  line L604 (-0.7839, 172.7853) -> (0, 172.5)
  line L605 (0, 172.5) -> (0.6366, 172.2683)
  line L606 (0.6366, 172.2683) -> (0.6366, 171.7317)
  line L607 (-0.7839, 172.7853) -> (-0.7839, 173)
  line L608 (-0.7839, 171.2147) -> (-0.7839, 171)
  line L609 (-0.7839, 173.2147) -> (0, 173.5)
  line L610 (0, 173.5) -> (0.6366, 173.7317)
  line L611 (-0.7839, 174.7853) -> (0, 174.5)
  line L612 (0, 174.5) -> (0.6366, 174.2683)
  line L613 (0.6366, 174.2683) -> (0.6366, 173.7317)
  line L614 (-0.7839, 174.7853) -> (-0.7839, 175)
  line L615 (-0.7839, 173.2147) -> (-0.7839, 173)
  line L616 (-0.7839, 175.2147) -> (0, 175.5)
  line L617 (0, 175.5) -> (0.6366, 175.7317)
  line L618 (-0.7839, 176.7853) -> (0, 176.5)
  line L619 (0, 176.5) -> (0.6366, 176.2683)
  line L620 (0.6366, 176.2683) -> (0.6366, 175.7317)
  line L621 (-0.7839, 176.7853) -> (-0.7839, 177)
  line L622 (-0.7839, 175.2147) -> (-0.7839, 175)
  line L623 (-0.7839, 177.2147) -> (0, 177.5)
  line L624 (0, 177.5) -> (0.6366, 177.7317)
  line L625 (-0.7839, 178.7853) -> (0, 178.5)
  line L626 (0, 178.5) -> (0.6366, 178.2683)
  line L627 (0.6366, 178.2683) -> (0.6366, 177.7317)
  line L628 (-0.7839, 178.7853) -> (-0.7839, 179)
  line L629 (-0.7839, 177.2147) -> (-0.7839, 177)
  line L630 (-0.7839, 179.2147) -> (0, 179.5)
  line L631 (0, 179.5) -> (0.6366, 179.7317)
  line L632 (-0.7839, 180.7853) -> (0, 180.5)
  line L633 (0, 180.5) -> (0.6366, 180.2683)
  line L634 (0.6366, 180.2683) -> (0.6366, 179.7317)
  line L635 (-0.7839, 180.7853) -> (-0.7839, 181)
  line L636 (-0.7839, 179.2147) -> (-0.7839, 179)
  line L637 (-0.7839, 181.2147) -> (0, 181.5)
  line L638 (0, 181.5) -> (0.6366, 181.7317)
  line L639 (-0.7839, 182.7853) -> (0, 182.5)
  line L640 (0, 182.5) -> (0.6366, 182.2683)
  line L641 (0.6366, 182.2683) -> (0.6366, 181.7317)
  line L642 (-0.7839, 182.7853) -> (-0.7839, 183)
  line L643 (-0.7839, 181.2147) -> (-0.7839, 181)
  line L644 (-0.7839, 183.2147) -> (0, 183.5)
  line L645 (0, 183.5) -> (0.6366, 183.7317)
  line L646 (-0.7839, 184.7853) -> (0, 184.5)
  line L647 (0, 184.5) -> (0.6366, 184.2683)
  line L648 (0.6366, 184.2683) -> (0.6366, 183.7317)
  line L649 (-0.7839, 184.7853) -> (-0.7839, 185)
  line L650 (-0.7839, 183.2147) -> (-0.7839, 183)
  line L651 (-0.7839, 185.2147) -> (0, 185.5)
  line L652 (0, 185.5) -> (0.6366, 185.7317)
  line L653 (-0.7839, 186.7853) -> (0, 186.5)
  line L654 (0, 186.5) -> (0.6366, 186.2683)
  line L655 (0.6366, 186.2683) -> (0.6366, 185.7317)
  line L656 (-0.7839, 186.7853) -> (-0.7839, 187)
  line L657 (-0.7839, 185.2147) -> (-0.7839, 185)
  line L658 (-0.7839, 187.2147) -> (0, 187.5)
  line L659 (0, 187.5) -> (0.6366, 187.7317)
  line L660 (-0.7839, 188.7853) -> (0, 188.5)
  line L661 (0, 188.5) -> (0.6366, 188.2683)
  line L662 (0.6366, 188.2683) -> (0.6366, 187.7317)
  line L663 (-0.7839, 188.7853) -> (-0.7839, 189)
  line L664 (-0.7839, 187.2147) -> (-0.7839, 187)
  line L665 (-0.7839, 189.2147) -> (0, 189.5)
  line L666 (0, 189.5) -> (0.6366, 189.7317)
  line L667 (-0.7839, 190.7853) -> (0, 190.5)
  line L668 (0, 190.5) -> (0.6366, 190.2683)
  line L669 (0.6366, 190.2683) -> (0.6366, 189.7317)
  line L670 (-0.7839, 190.7853) -> (-0.7839, 191)
  line L671 (-0.7839, 189.2147) -> (-0.7839, 189)
  line L672 (-0.7839, -1) -> (-5.7839, -1)
  line L673 (-5.7839, -1) -> (-5.7839, 189)
  line L674 (-5.7839, 189) -> (-0.7839, 189)
extrude "Extrude1'" add sketch "Sketch1 (2)" along normal blind 2.5 and the other way blind 2.5 separate body makes body 2 in component "Rack; Circular Pitch: 2.00 mm; Num Teeth: 95; Pressure Angle: 20 deg; Backlash: 0.00 mm;"
sketch "Sketch2 (2)" plane through (0, 0, 0) normal (0, 0, 1) x (1, 0, 0) in component "Rack; Circular Pitch: 2.00 mm; Num Teeth: 95; Pressure Angle: 20 deg; Backlash: 0.00 mm;"
  line L0 (0, 0) -> (0, 188) construction
sketch "Sketch5" plane through (0, 0, 5) normal (0, 0, 1) x (1, 0, 0)
  line L0 (152.4, 0) -> (152.4, 101.6)
  line L1 (152.4, 101.6) -> (0, 101.6)
  line L2 (0, 101.6) -> (0, 0)
  line L3 (0, 0) -> (25, 0)
  line L4 (25, 0) -> (25, 15)
  line L5 (25, 15) -> (127.4, 15)
  line L6 (127.4, 15) -> (127.4, 0)
  line L7 (127.4, 0) -> (152.4, 0)
  line L8 (0, 101.6) -> (0, 86.6)
  line L9 (152.4, 101.6) -> (152.4, 86.6)
  line L10 (152.4, 101.6) -> (142.4, 101.6)
  line L11 (142.4, 101.6) -> (142.4, 91.6)
  line L12 (142.4, 91.6) -> (152.4, 91.6)
  line L13 (152.4, 91.6) -> (152.4, 101.6)
  circle A0 centre (142.4, 91.6) radius 5.343
  line L14 (0, 101.6) -> (10, 101.6)
  line L15 (10, 101.6) -> (10, 91.6)
  line L16 (10, 91.6) -> (0, 91.6)
  line L17 (0, 91.6) -> (0, 101.6)
  circle A1 centre (10, 91.6) radius 5.343
  line L18 (0, 101.6) -> (25, 101.6)
  line L19 (152.4, 101.6) -> (127.4, 101.6)
  line L20 (25, 101.6) -> (127.4, 101.6)
  line L21 (127.4, 101.6) -> (127.4, 59.6)
  line L22 (127.4, 59.6) -> (25, 59.6)
  line L23 (25, 59.6) -> (25, 101.6)
  dimension "d39" = 15
  dimension "d45" = 10
  dimension "d46" = 10
  dimension "d47" = 10.686
  dimension "d48" = 10
  dimension "d49" = 10
  dimension "d50" = 10.686
  dimension "d51" = 25
  dimension "d52" = 102.4
  dimension "d53" = 42
  constraint coincident L1.end L2.start
  constraint perpendicular L1 L8
  constraint coincident L0.end L1.start
  constraint perpendicular L1 L9
  constraint horizontal L10
  constraint vertical L11
  constraint horizontal L12
  constraint vertical L13
  constraint coincident L11.end L12.start
  constraint horizontal L14
  constraint vertical L15
  constraint horizontal L16
  constraint vertical L17
  constraint coincident L15.end L16.start
  constraint coincident L1 L18.end
  constraint perpendicular L17 L18
  constraint perpendicular L9 L19
  constraint horizontal L20
  constraint vertical L21
  constraint horizontal L22
  constraint vertical L23
  measures "d39" distance of L1.end L8.end
  measures "d45" distance of L0.end L10.end
  measures "d46" distance of L0.end L12.end
  measures "d47" diameter of A0
  measures "d48" distance of L1.end L14.end
  measures "d49" distance of L1.end L16.end
  measures "d50" diameter of A1
  measures "d51" distance of L0.end L19.end
  measures "d52" distance of L18.end L19.end
  measures "d53" distance of L18.end L22.end
extrude "Extrude4" cut sketch "Sketch5" against normal blind 5 contours L11 L12 A0 | L11 L12 A0 | L1 L20 L21 L22 L23 | L15 L16 A1 | L15 L16 A1 bodies 1
sketch "Sketch6" plane through (0, 0, -198.04) normal (0, 0, -1) x (-1, 0, 0)
  line L0 (-25, 15) -> (-25, 0)
  line L1 (-25, 0) -> (-0.3217, 0)
  line L2 (-0.3217, 0) -> (-0.3217, 101.3242)
  line L3 (-0.3217, 101.3242) -> (-152.4, 101.3242)
  line L4 (-152.4, 101.3242) -> (-152.4, 0)
  line L5 (-152.4, 0) -> (-127.4, 0)
  line L6 (-127.4, 0) -> (-127.4, 15)
  line L7 (-127.4, 15) -> (-25, 15)
  line L8 (-152.4, 101.3242) -> (-142.4, 101.3242)
  line L9 (-142.4, 101.3242) -> (-142.4, 91.3242)
  line L10 (-142.4, 91.3242) -> (-152.4, 91.3242)
  line L11 (-152.4, 91.3242) -> (-152.4, 101.3242)
  line L12 (-0.3217, 101.3242) -> (-10.3217, 101.3242)
  line L13 (-10.3217, 101.3242) -> (-10.3217, 91.3242)
  line L14 (-10.3217, 91.3242) -> (-0.3217, 91.3242)
  line L15 (-0.3217, 91.3242) -> (-0.3217, 101.3242)
  circle A0 centre (-142.4, 91.3242) radius 5.334
  circle A1 centre (-10.3217, 91.3242) radius 5.343
  line L16 (-152.4, 101.3242) -> (-127.4, 101.3242)
  line L17 (-127.4, 101.3242) -> (-127.4, 59.3242)
  line L18 (-127.4, 59.3242) -> (-152.4, 59.3242)
  line L19 (-152.4, 59.3242) -> (-152.4, 101.3242)
  line L20 (-0.3217, 101.3242) -> (-25.3217, 101.3242)
  line L21 (-25.3217, 101.3242) -> (-25.3217, 59.3242)
  line L22 (-25.3217, 59.3242) -> (-0.3217, 59.3242)
  line L23 (-0.3217, 59.3242) -> (-0.3217, 101.3242)
  line L24 (-127.4, 59.3242) -> (-25.3217, 59.3242)
  line L25 (-25.3217, 59.3242) -> (-25.3217, 101.3242)
  line L26 (-25.3217, 101.3242) -> (-127.4, 101.3242)
  line L27 (-127.4, 101.3242) -> (-127.4, 59.3242)
  dimension "d58" = 10
  dimension "d59" = 10
  dimension "d60" = 10
  dimension "d61" = 10
  dimension "d62" = 10.668
  dimension "d63" = 10.686
  dimension "d64" = 25
  dimension "d65" = 42
  dimension "d66" = 25
  dimension "d67" = 42
  constraint horizontal L8
  constraint vertical L9
  constraint horizontal L10
  constraint vertical L11
  constraint coincident L3.end L4.start
  constraint horizontal L12
  constraint vertical L13
  constraint horizontal L14
  constraint vertical L15
  constraint coincident L2.end L3.start
  constraint coincident L9.end L10.start
  constraint coincident L13.end L14.start
  constraint horizontal L16
  constraint vertical L17
  constraint horizontal L18
  constraint vertical L19
  constraint horizontal L20
  constraint vertical L21
  constraint horizontal L22
  constraint vertical L23
  constraint horizontal L24
  constraint vertical L25
  constraint horizontal L26
  constraint vertical L27
  measures "d58" distance of L3.end L8.end
  measures "d59" distance of L3.end L10.end
  measures "d60" distance of L2.end L12.end
  measures "d61" distance of L2.end L14.end
  measures "d62" diameter of A0
  measures "d63" diameter of A1
  measures "d64" distance of L3.end L16.end
  measures "d65" distance of L3.end L18.end
  measures "d66" distance of L2.end L20.end
  measures "d67" distance of L2.end L22.end
extrude "Extrude5" cut sketch "Sketch6" against normal blind 5 contours L3 L17 L21 L24 L25 L26 L27 | L13 L14 A1 | L13 L14 A1 | L9 L10 A0 | L9 L10 A0 bodies 1
sketch "Sketch7" plane through (0, 0, 0) normal (-1, 0, 0) x (0, 0, 1)
  line L0 (0, 101.6) -> (0, 65)
  line L1 (0, 65) -> (-193.04, 65)
  line L2 (-193.04, 65) -> (-193.04, 0)
  line L3 (-193.04, 0) -> (5, 0)
  line L4 (5, 0) -> (5, 101.6)
  line L5 (5, 101.6) -> (0, 101.6)
component "Rack; Circular Pitch: 2.00 mm; Num Teeth: 95; Pressure Angle: 20 deg; Backlash: 0.00 mm;" placed x (0, 1, 0) y (0, 0, -1) z (-1, 0, 0) at (3.5, 70.7839, -2)
